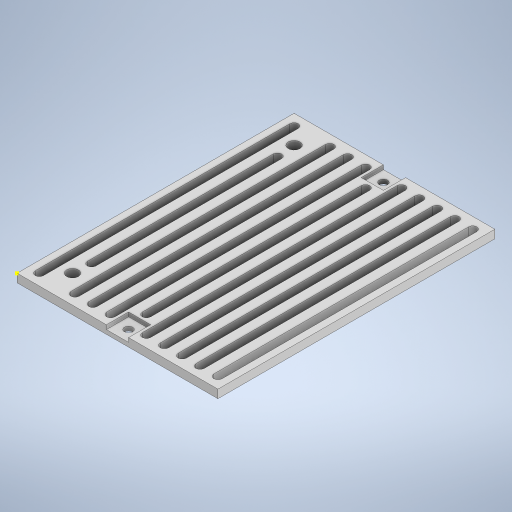
# Autodesk Inventor part: Tray
Saved by Autodesk Inventor 2024 (Build 280153000, 153)
## iProperties
Created: 2023-11-19
Part Number: Tray
Material: Generic
Document SubType Name: Modeling
Designer: olson
Density: 1 g/cm^3
Appearance: Default
Author: olson
Autodesk Inventor part; units mm, degrees
ref_plane "YZ Plane" through (0, 0, 0) normal (1, 0, 0) x (0, 1, 0)
ref_plane "XZ Plane" through (0, 0, 0) normal (0, 1, 0) x (-1, 0, 0)
ref_plane "XY Plane" through (0, 0, 0) normal (0, 0, 1) x (1, 0, 0)
sketch "Sketch1" plane through (0, 0, 0) normal (0, 1, 0) x (-1, 0, 0)
  line L0 (0, 0) -> (-72.5, 0)
  line L1 (-72.5, 0) -> (-72.5, -100)
  line L2 (-72.5, -100) -> (0, -100)
  line L3 (0, -100) -> (0, 0)
  dimension "d0" = 72.5
  dimension "d1" = 100
  constraints: 8 end point, 2 parallel, 1 horizontal, 1 perpendicular
  measures "d0" distance of L2.end L1.end
  measures "d1" distance of L1.end L0.end
extrude "Extrusion1" add sketch "Sketch1" along normal blind 3
sketch "Sketch7" plane through (0, 3, 0) normal (0, 1, 0) x (1, 0, 0)
  line L0 (72.5, 100) -> (0, 100) projected
  line L1 (0, 0) -> (72.5, 0)
  line L2 (72.5, 0) -> (72.5, 100)
  line L3 (72.5, 100) -> (0, 100)
  line L4 (0, 100) -> (0, 0)
  line L5 (0, 0) -> (0, 9.525)
  line L6 (0, 0) -> (10, 0)
  line L7 (10, 0) -> (10, 10)
  line L8 (10, 10) -> (0, 10)
  line L9 (0, 10) -> (0, 0)
  line L10 (0, 100) -> (10, 100)
  line L11 (10, 100) -> (10, 90)
  line L12 (10, 90) -> (0, 90)
  line L13 (0, 90) -> (0, 100)
  line L14 (72.5, 100) -> (62.5, 100)
  line L15 (62.5, 100) -> (62.5, 90)
  line L16 (62.5, 90) -> (72.5, 90)
  line L17 (72.5, 90) -> (72.5, 100)
  circle A0 centre (95, 95) radius 1.5
  line L18 (72.5, 0) -> (62.5, 0)
  line L19 (62.5, 0) -> (62.5, 10)
  line L20 (62.5, 10) -> (72.5, 10)
  line L21 (72.5, 10) -> (72.5, 0)
  circle A1 centre (95, 5) radius 1.5
  circle A2 centre (10, 90) radius 2.125
  circle A3 centre (10, 10) radius 2.125
  point P0 (41.25, 100)
  dimension "d36" = 10
  dimension "d37" = 10
  dimension "d39" = 10
  dimension "d40" = 10
  dimension "d42" = 10
  dimension "d43" = 10
  dimension "d44" = 3
  dimension "d45" = 10
  dimension "d46" = 10
  dimension "d47" = 3
  dimension "d181" = 4.25
  dimension "d182" = 4.25
  constraints: 42 end point, 10 parallel, 5 horizontal, 5 perpendicular, 4 centre point, 2 coincident, 1 point on line
  measures "d36" distance of L8.end L7.end
  measures "d37" distance of L7.end L6.end
  measures "d39" distance of L11.end L12.end
  measures "d40" distance of L10.end L11.end
  measures "d42" distance of L16.end L15.end
  measures "d43" distance of L15.end L14.end
  measures "d44" diameter of A0
  measures "d45" distance of L19.end L20.end
  measures "d46" distance of L18.end L19.end
  measures "d47" diameter of A1
  measures "d181" diameter of A2
  measures "d182" diameter of A3
extrude "Extrusion7" cut sketch "Sketch7" against normal blind 3 contours A2 L12 L11 | L11 L12 A2 | A3 L7 L8 | L8 L7 A3 | A0 | A1
sketch "Sketch11" plane through (0, 3, 0) normal (0, 1, 0) x (1, 0, 0)
  point P0 (0, 0)
sketch "Sketch13" plane through (0, 3, 0) normal (0, 1, 0) x (1, 0, 0)
  line L0 (0, 0) -> (72.5, 0) projected
  line L1 (36.25, 0) -> (36.25, 8)
  line L2 (36.25, 8) -> (32.25, 8)
  line L3 (32.25, 8) -> (32.25, 0)
  line L4 (36.25, 0) -> (32.25, 0)
  line L5 (36.25, 0) -> (40.25, 0)
  line L6 (40.25, 0) -> (40.25, 8)
  line L7 (40.25, 8) -> (36.25, 8)
  line L8 (72.5, 100) -> (0, 100) projected
  line L9 (36.25, 100) -> (32.25, 100)
  line L10 (32.25, 100) -> (32.25, 92)
  line L11 (32.25, 92) -> (40.25, 92)
  line L12 (40.25, 92) -> (40.25, 100)
  line L13 (40.25, 100) -> (36.25, 100)
  line L14 (72.5, 0) -> (72.5, 100) projected
  dimension "d190" = 8
  dimension "d191" = 4
  dimension "d192" = 4
  dimension "d193" = 8
  constraints: 24 end point, 9 point on line, 5 perpendicular, 2 midpoint, 1 collinear, 1 horizontal, 1 vertical
  measures "d190" distance of L1.start L1.end
  measures "d191" distance of L1.end L2.end
  measures "d192" distance of L1.start L5.end
  measures "d193" distance of L9.end L10.end
extrude "Extrusion11" cut sketch "Sketch13" against normal blind 1.5
sketch "Sketch14" plane through (0, 1.5, 0) normal (0, 1, 0) x (1, 0, 0)
  line L0 (0, 0) -> (72.5, 0) projected
  line L1 (40.25, 8) -> (32.25, 8)
  line L2 (32.25, 8) -> (32.25, 0)
  line L3 (32.25, 0) -> (40.25, 0)
  line L4 (40.25, 0) -> (40.25, 8)
  line L5 (72.5, 100) -> (0, 100) projected
  line L6 (40.25, 100) -> (32.25, 100)
  line L7 (32.25, 100) -> (32.25, 92)
  line L8 (32.25, 92) -> (40.25, 92)
  line L9 (40.25, 92) -> (40.25, 100)
  circle A0 centre (36.25, 4) radius 1.5
  circle A1 centre (36.25, 96) radius 1.5
  point P0 (72.5, 46)
  point P1 (64.5, 54)
  dimension "d199" = 8
  dimension "d200" = 8
  dimension "d201" = 3
  dimension "d202" = 3
  constraints: 16 end point, 4 parallel, 4 point on line, 2 centre point, 2 horizontal, 2 perpendicular
  measures "d199" distance of L3.end L2.end
  measures "d200" distance of L7.end L6.end
  measures "d201" diameter of A0
  measures "d202" diameter of A1
extrude "Extrusion12" cut sketch "Sketch14" against normal blind 1.5 contours A0 | A1
sketch "Sketch15" plane through (0, 3, 0) normal (0, 1, 0) x (1, 0, 0)
  circle A0 centre (36.25, 4) radius 1.5 projected
  line L0 (0, 100) -> (0, 0) projected
  circle A1 centre (36.25, 96) radius 1.5 projected
  line L1 (32.25, 8) -> (40.25, 8) projected
  arc A2 (2.5, 4) -> (5.5, 4) centre (4, 4) ccw
  arc A3 (15.4, 4) -> (18.4, 4) centre (16.9, 4) ccw
  arc A4 (21.85, 4) -> (24.85, 4) centre (23.35, 4) ccw
  arc A5 (28.3, 4) -> (31.3, 4) centre (29.8, 4) ccw
  arc A6 (41.2, 4) -> (44.2, 4) centre (42.7, 4) ccw
  arc A7 (47.65, 4) -> (50.65, 4) centre (49.15, 4) ccw
  arc A8 (54.1, 4) -> (57.1, 4) centre (55.6, 4) ccw
  arc A9 (60.55, 4) -> (63.55, 4) centre (62.05, 4) ccw
  arc A10 (67, 4) -> (70, 4) centre (68.5, 4) ccw
  arc A11 (70, 96) -> (67, 96) centre (68.5, 96) ccw
  arc A12 (63.55, 96) -> (60.55, 96) centre (62.05, 96) ccw
  arc A13 (57.1, 96) -> (54.1, 96) centre (55.6, 96) ccw
  arc A14 (50.65, 96) -> (47.65, 96) centre (49.15, 96) ccw
  arc A15 (44.2, 96) -> (41.2, 96) centre (42.7, 96) ccw
  arc A16 (31.3, 96) -> (28.3, 96) centre (29.8, 96) ccw
  arc A17 (24.85, 96) -> (21.85, 96) centre (23.35, 96) ccw
  arc A18 (18.4, 96) -> (15.4, 96) centre (16.9, 96) ccw
  arc A19 (5.5, 96) -> (2.5, 96) centre (4, 96) ccw
  circle A20 centre (10, 90) radius 2.125 projected
  line L2 (10, 90) -> (10.45, 90)
  line L3 (10.45, 90) -> (10.45, 83.55)
  arc A21 (11.95, 83.55) -> (8.95, 83.55) centre (10.45, 83.55) ccw
  circle A22 centre (10, 10) radius 2.125 projected
  line L4 (10, 10) -> (10.45, 10)
  line L5 (10.45, 10) -> (10.45, 16.45)
  arc A23 (8.95, 16.45) -> (11.95, 16.45) centre (10.45, 16.45) ccw
  line L6 (5.5, 4) -> (5.5, 96)
  line L7 (2.5, 96) -> (2.5, 4)
  line L8 (8.95, 16.45) -> (8.95, 83.55)
  line L9 (11.95, 83.55) -> (11.95, 16.45)
  line L10 (15.4, 4) -> (15.4, 96)
  line L11 (18.4, 96) -> (18.4, 4)
  line L12 (21.85, 96) -> (21.85, 4)
  line L13 (24.85, 4) -> (24.85, 96)
  line L14 (28.3, 96) -> (28.3, 4)
  line L15 (31.3, 4) -> (31.3, 96)
  line L16 (41.2, 96) -> (41.2, 4)
  line L17 (44.2, 4) -> (44.2, 96)
  line L18 (47.65, 96) -> (47.65, 4)
  line L19 (50.65, 4) -> (50.65, 96)
  line L20 (54.1, 96) -> (54.1, 4)
  line L21 (57.1, 4) -> (57.1, 96)
  line L22 (60.55, 96) -> (60.55, 4)
  line L23 (63.55, 4) -> (63.55, 96)
  line L24 (67, 43.55) -> (67, 4)
  line L25 (70, 4) -> (70, 43.55)
  line L26 (67, 56.45) -> (67, 96)
  line L27 (70, 96) -> (70, 56.45)
  line L28 (36.25, 4) -> (36.25, 10.45)
  arc A24 (34.75, 10.45) -> (37.75, 10.45) centre (36.25, 10.45) ccw
  line L29 (36.25, 96) -> (36.25, 89.55)
  arc A25 (37.75, 89.55) -> (34.75, 89.55) centre (36.25, 89.55) ccw
  line L30 (34.75, 10.45) -> (34.75, 89.55)
  line L31 (37.75, 89.55) -> (37.75, 10.45)
  line L32 (67, 56.45) -> (67, 43.55)
  line L33 (70, 43.55) -> (70, 56.45)
  dimension "d216" = 3
  dimension "d217" = 3
  dimension "d218" = 3
  dimension "d219" = 3
  dimension "d220" = 3
  dimension "d221" = 3
  dimension "d225" = 3
  dimension "d226" = 3
  dimension "d227" = 3
  dimension "d228" = 3
  dimension "d229" = 3
  dimension "d230" = 3
  dimension "d231" = 3
  dimension "d232" = 3
  dimension "d233" = 3
  dimension "d234" = 6.45
  dimension "d235" = 3
  dimension "d236" = 6.45
  dimension "d237" = 3
  dimension "d242" = 6.45
  dimension "d243" = 3
  dimension "d244" = 6.45
  dimension "d245" = 3
  constraints: 64 end point, 44 point on circle, 22 centre point, 21 tangent, 4 coincident, 4 parallel, 4 point on line, 2 vertical, 1 collinear
  measures "d216" diameter of A2
  measures "d217" diameter of A3
  measures "d218" diameter of A4
  measures "d219" diameter of A5
  measures "d220" diameter of A6
  measures "d221" diameter of A7
  measures "d225" diameter of A11
  measures "d226" diameter of A12
  measures "d227" diameter of A13
  measures "d228" diameter of A14
  measures "d229" diameter of A15
  measures "d230" diameter of A16
  measures "d231" diameter of A17
  measures "d232" diameter of A18
  measures "d233" diameter of A19
  measures "d234" distance of L2.end L3.end
  measures "d235" diameter of A21
  measures "d236" distance of L4.end L5.end
  measures "d237" diameter of A23
  measures "d242" distance of L28.start L28.end
  measures "d243" diameter of A24
  measures "d244" distance of L29.start L29.end
  measures "d245" diameter of A25
extrude "Extrusion13" cut sketch "Sketch15" against normal blind 3 contours A24 L30 A25 L31 | L7 A19 L6 A2 | L10 A18 L11 A3 | L12 A17 L13 A4 | L14 A16 L15 A5 | L16 A15 L17 A6 | L18 A14 L19 A7 | L20 A13 L21 A8 | L22 A12 L23 A9 | L24 L32 L26 A11 L27 L33 L25 A10 | A21 L9 A23 L8
sketch "Sketch16" plane through (0, 3, 0) normal (0, 1, 0) x (1, 0, 0)
  point P0 (0, 0)
body "Solid1"
